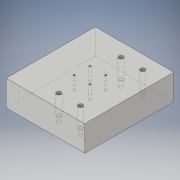
# Autodesk Inventor part: Chuck Spacer
Saved by Autodesk Inventor 2019.4 (Build 234330000, 330)
## iProperties
Created: 2021-01-20
Part Number: Chuck Spacer
Material: Generic
Document SubType Name: Modeling
Designer: caleb
Density: 1 g/cm^3
Appearance: Default
Author: caleb
Autodesk Inventor part; units mm, degrees
ref_plane "YZ Plane" through (0, 0, 0) normal (1, 0, 0) x (0, 1, 0)
ref_plane "XZ Plane" through (0, 0, 0) normal (0, 1, 0) x (-1, 0, 0)
ref_plane "XY Plane" through (0, 0, 0) normal (0, 0, 1) x (1, 0, 0)
sketch "Sketch1" plane through (0, 0, 0) normal (0, 1, 0) x (-1, 0, 0)
  line L0 (-75, 85) -> (75, 85)
  line L1 (75, 85) -> (75, -85)
  line L2 (75, -85) -> (-75, -85)
  line L3 (-75, -85) -> (-75, 85)
  line L4 (-75, 85) -> (75, -85) construction
  line L5 (75, 85) -> (-75, -85) construction
  point P0 (0, 0)
  dimension "d0" = 170
  dimension "d1" = 150
  constraints: 12 end point, 2 midpoint, 2 parallel, 1 horizontal, 1 perpendicular
  measures "d0" distance of L0.end L1.end
  measures "d1" distance of L1.end L2.end
extrude "Extrusion1" add sketch "Sketch1" along normal blind 48.768
sketch "Sketch2" plane through (0, 48.768, 0) normal (0, 1, 0) x (1, 0, 0)
  line L0 (75, 85) -> (-75, 85) projected
  line L1 (-75, 85) -> (-75, -85) projected
  point P0 (0, 0)
  point P1 (-15, 15)
  point P2 (15, 15)
  point P3 (-15, -15)
  point P4 (15, -15)
  dimension "d4" = 15
  dimension "d5" = 15
  dimension "d8" = 30
  dimension "d11" = 30
  constraints: 1 horizontal, 1 vertical, 3 other
  measures "d4" horizontal distance of point (0, 0) point (-15, 15)
  measures "d5" horizontal distance of point (-15, 15) point (0, 0)
  measures "d8" distance of point (-15, 15) point (15, 15)
  measures "d11" distance of point (-15, 15) point (-15, -15)
hole "Hole1" at (-15, 48.768, -15) at (15, 48.768, -15) at (-15, 48.768, 15) at (15, 48.768, 15) direction (0, -1, 0) diameter 3.242 depth 25.4 tip angle 118 thread size "M4x0.7" class "6H" standard "ANSI Metric M Profile"
sketch "Sketch3" plane through (0, 48.768, 0) normal (0, 1, 0) x (1, 0, 0)
  line L0 (-75, -85) -> (75, -85) projected
  line L1 (75, -85) -> (75, 85) projected
  point P0 (0, 0)
  point P1 (41.2688, -59.2952)
  point P2 (41.2688, 59.3228)
  point P3 (-0.0062, -59.2952)
  point P4 (-0.0062, 59.3228)
  dimension "d21" = 25.7048
  dimension "d22" = 33.7312
  dimension "d25" = 118.618
  dimension "d28" = 41.275
  constraints: 1 horizontal, 1 vertical, 3 other
  measures "d21" distance from line of L0 point (41.269, -59.295)
  measures "d22" distance from line of L1 point (41.269, -59.295)
  measures "d25" distance of point (41.269, -59.295) point (41.269, 59.323)
  measures "d28" distance of point (41.269, -59.295) point (-0.006, -59.295)
hole "Hole2" at (41.2688, 48.768, 59.2952) at (41.2688, 48.768, -59.3228) at (-0.0062, 48.768, 59.2952) at (-0.0062, 48.768, -59.3228) direction (0, -1, 0) diameter 6.756 end through all counterbore diameter 8.636 counterbore depth 36.83 clearance for "Hex Head Bolt" size "1/4" standard "Ansi Unified Screw Threads"
body "Solid1"
